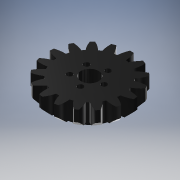
# Autodesk Inventor part: Spur Gear1
Saved by Autodesk Inventor 2017 (Build 210142000, 142)
## iProperties
Created: 2019-10-27
Part Number: Spur Gear1
Material: ABS Plastic
Document SubType Name: Modeling
Designer: Zach
Categories: <?xml version="1.0" encoding="UTF-16"?> <MemberInstance><Categories><FamilyTemplate><FamilyTemplateParameter ValueType="xs:double" Id="1" ObjectReferenceKey="da_z" ObjectType="kUserParameterObject"/><FamilyTemplateParameter ValueType="xs:double" Id="2" ObjectReferenceKey="da_b" ObjectType="kUserParameterObject"/><FamilyTemplateParameter ValueType="xs:double" Id="3" ObjectReferenceKey="da_beta" ObjectType="kUserParameterObject"/><FamilyTemplateParameter ValueType="xs:double" Id="4" ObjectReferenceKey="da_da" ObjectType="kUserParameterObject"/><FamilyTemplateParameter ValueType="xs:double" Id="5" ObjectReferenceKey="da_aw" ObjectType="kUserParameterObject"/><FamilyTemplateParameter ValueType="xs:string" Id="6" ObjectReferenceKey="EAIAABAAAACIAQAAAAAAAIAAAAAAAAAA" ObjectType="83910656" SubObjectId="SurfaceGeometry"/></FamilyTemplate><ParamToTemplateMap><ParamToTemplate CategoryParameter="//CategoryParameter[@InternalName='046C89C9-8512-4d59-83FE-43B91F4F132A']" TemplateParameter="1"/><ParamToTemplate CategoryParameter="//CategoryParameter[@InternalName='2552DF32-E462-4b46-AEBF-C6C7768E72AC']" TemplateParameter="2"/><ParamToTemplate CategoryParameter="//CategoryParameter[@InternalName='C9EE641D-15FC-4fae-A226-E94C4372FDD7']" TemplateParameter="3"/><ParamToTemplate><ParamToTemplate CategoryParameter="//CategoryParameter[@InternalName='00B6519A-459B-49c7-AD84-2E56D39A5744']" ConstantValue="0.000000"/></ParamToTemplate><ParamToTemplate><ParamToTemplate CategoryParameter="//CategoryParameter[@InternalName='04B31F0E-C7A6-4894-AA32-9629BEFACF47']" ConstantValue="1.000000"/></ParamToTemplate><ParamToTemplate><ParamToTemplate CategoryParameter="//CategoryParameter[@InternalName='43CBEC2E-7847-49e7-A936-2F7889FCB2D9']" ConstantValue="0.250000"/></ParamToTemplate><ParamToTemplate><ParamToTemplate CategoryParameter="//CategoryParameter[@InternalName='B1EFC894-105D-4ebd-86BF-FA20ED196853']" ConstantValue="0.350000"/></ParamToTemplate><ParamToTemplate><ParamToTemplate CategoryParameter="//CategoryParameter[@InternalName='51175063-3D10-4879-93E8-6246FE8B403D']" ConstantValue="2060000000.000000"/></ParamToTemplate><ParamToTemplate><ParamToTemplate CategoryParameter="//CategoryParameter[@InternalName='A3A52E27-4454-46a9-B0BD-C932399B70AF']" ConstantValue="0.300000"/></ParamToTemplate><ParamToTemplate><ParamToTemplate CategoryParameter="//CategoryParameter[@InternalName='91B76062-C214-41d9-B1B9-14D2AB99603D']" ConstantValue="0.200000"/></ParamToTemplate><ParamToTemplate><ParamToTemplate CategoryParameter="//CategoryParameter[@InternalName='374E806E-8B8A-4dda-A9AA-1039D6500AD2']" ConstantValue="5.000000"/></ParamToTemplate><ParamToTemplate><ParamToTemplate CategoryParameter="//CategoryParameter[@InternalName='2D373A89-B862-43d6-8D0B-0CBF12AB9F6C']" ConstantValue="0.392699"/></ParamToTemplate><ParamToTemplate CategoryParameter="//CategoryParameter[@InternalName='37777632-D6A2-4fac-9D53-DB8ACD95C989']" TemplateParameter="4"/><ParamToTemplate CategoryParameter="//CategoryParameter[@InternalName='FD1017F1-B727-4f7e-9707-0F86F1FF9423']" TemplateParameter="5"/><ParamToTemplate><ParamToTemplate CategoryParameter="//CategoryParameter[@InternalName='9E1B4470-B2D3-4ff1-B813-535BB4CDF51A']" ConstantValue="3520000.000000"/></ParamToTemplate><ParamToTemplate><ParamToTemplate CategoryParameter="//CategoryParameter[@InternalName='F8452263-BFF6-458c-9FB1-07C4B99E95CD']" ConstantValue="11400000.000000"/></ParamToTemplate><ParamToTemplate><ParamToTemplate CategoryParameter="//CategoryParameter[@InternalName='3E3BB259-FD49-497f-8171-6EBC954A3479']" ConstantValue="2.000000"/></ParamToTemplate><ParamToTemplate CategoryParameter="//CategoryParameter[@InternalName='27C3BAF2-7550-4e4b-AE2C-0DB134B7D9B7']" TemplateParameter="6"/></ParamToTemplateMap><Category DisplayName="Gear" InternalName="DC85795E-93AB-48d5-8EEE-5A27447B64BD" Mnemonic="Gear"><CategoryParameter DisplayName="z" InternalName="046C89C9-8512-4d59-83FE-43B91F4F132A" Mnemonic="z"/><CategoryParameter DisplayName="b" InternalName="2552DF32-E462-4b46-AEBF-C6C7768E72AC" Mnemonic="b"/><CategoryParameter DisplayName="||b|" InternalName="C9EE641D-15FC-4fae-A226-E94C4372FDD7" Mnemonic="beta"/><CategoryParameter DisplayName="x" InternalName="00B6519A-459B-49c7-AD84-2E56D39A5744" Mnemonic="x"/><CategoryParameter DisplayName="a*" InternalName="04B31F0E-C7A6-4894-AA32-9629BEFACF47" Mnemonic="a"/><CategoryParameter DisplayName="c*" InternalName="43CBEC2E-7847-49e7-A936-2F7889FCB2D9" Mnemonic="c"/><CategoryParameter DisplayName="r|.f|*" InternalName="B1EFC894-105D-4ebd-86BF-FA20ED196853" Mnemonic="rf"/><CategoryParameter DisplayName="E" InternalName="51175063-3D10-4879-93E8-6246FE8B403D" Mnemonic="E"/><CategoryParameter DisplayName="||m|" InternalName="A3A52E27-4454-46a9-B0BD-C932399B70AF" Mnemonic="mi"/><Category DisplayName="SpurGear" InternalName="26C5A22E-A91E-4dfd-A3B3-23CCAFAE1764" Mnemonic="SpurGear"><CategoryParameter DisplayName="m" InternalName="91B76062-C214-41d9-B1B9-14D2AB99603D" Mnemonic="m"/><CategoryParameter DisplayName="P" InternalName="374E806E-8B8A-4dda-A9AA-1039D6500AD2" Mnemonic="PP"/><CategoryParameter DisplayName="||a|" InternalName="2D373A89-B862-43d6-8D0B-0CBF12AB9F6C" Mnemonic="alpha"/><CategoryParameter DisplayName="d|.a|" InternalName="37777632-D6A2-4fac-9D53-DB8ACD95C989" Mnemonic="da"/><CategoryParameter DisplayName="a|.w|" InternalName="FD1017F1-B727-4f7e-9707-0F86F1FF9423" Mnemonic="aw"/><CategoryParameter DisplayName="||s||.Flim|" InternalName="9E1B4470-B2D3-4ff1-B813-535BB4CDF51A" Mnemonic="sFlim"/><CategoryParameter DisplayName="||s||.Hlim|" InternalName="F8452263-BFF6-458c-9FB1-07C4B99E95CD" Mnemonic="sHlim"/><CategoryParameter DisplayName="type" InternalName="3E3BB259-FD49-497f-8171-6EBC954A3479" Mnemonic="type"/><CategoryParameter DisplayName="PitchDiameter" InternalName="27C3BAF2-7550-4e4b-AE2C-0DB134B7D9B7" Mnemonic="IDS_PITCHDIAM"/></Category></Category></Categories></MemberInstance>
Density: 1.06 g/cm^3
Appearance: Smooth - Black
CustomPartVersion: 1
Author: Zach
Autodesk Inventor part; units mm, degrees
sketch "Sketch1" plane through (0, 0, 0) normal (0, 0, 1) x (1, 0, 0)
  circle A0 centre (0, 0) radius 19
  dimension "d0" = 38
  constraints: 1 centre point
  measures "d0" diameter of A0
extrude "Extrusion1" add sketch "Sketch1" along normal blind 8
ref_plane "Work Plane2" through (0, 0, 4) normal (0, 0, 1) x (1, 0, 0)
sketch "Sketch2" plane through (0, 0, 0) normal (0, 0, -1) x (-1, 0, 0)
  circle A0 centre (0, 0) radius 19 projected
  circle A1 centre (0, 0) radius 17
  dimension "d3" = 34
  constraints: 1 centre point, 1 coincident
  measures "d3" diameter of A1
surface extrude "Pitch Diameter" sketch "Sketch2" against normal through all shown no curves A1
ref_plane "Work Plane8" through (0, 0, 0) normal (0.9829731, 0.1837495, 0) x (0, 0, 1)
ref_plane "Work Plane9" through (0, 0, 0) normal (1, 0, 0) x (0, 1, 0)
spur gear teeth "Spur Gear" teeth 17 pitch diameter 34 tip diameter 38 root diameter 29 face width 8 start plane through (0, 0, 0) normal (0, 0, -1) x (-1, 0, 0)
sketch "Sketch3" plane through (0, 0, 8) normal (0, 0, 1) x (1, 0, 0)
  circle A0 centre (0, 0) radius 4
  circle A1 centre (6.5, 0) radius 1.25
  circle A2 centre (2.0086, 6.1819) radius 1.25
  circle A3 centre (-5.2586, 3.8206) radius 1.25
  circle A4 centre (-5.2586, -3.8206) radius 1.25
  circle A5 centre (2.0086, -6.1819) radius 1.25
  dimension "d49" = 8
  dimension "d50" = 2.5
  dimension "d51" = 6.5
  dimension "d54" = 360
  constraints: 6 centre point, 1 coincident, 1 horizontal alignment, 11 other
  measures "d49" diameter of A0
  measures "d50" diameter of A1
  measures "d51" distance of A1.centre point (0, 0)
extrude "Extrusion2" cut sketch "Sketch3" against normal through all
sketch "Sketch4" plane through (0, 0, 0) normal (0, 0, -1) x (-1, 0, 0)
  circle A0 centre (0, 0) radius 11.5
  circle A1 centre (-2.0086, -6.1819) radius 1.25 projected
  circle A2 centre (5.2586, 3.8206) radius 1.25 projected
  circle A3 centre (-6.5, 0) radius 1.25 projected
  circle A4 centre (-2.0086, 6.1819) radius 1.25 projected
  circle A5 centre (5.2586, -3.8206) radius 1.25 projected
  circle A6 centre (0, 0) radius 4 projected
  arc A7 (0.8775, 18.9797) -> (-0.8775, 18.9797) centre (0, 0) ccw projected
  arc A8 (6.038, 18.0151) -> (3.3198, 14.1149) centre (16.9951, 7.4811) ccw projected
  arc A9 (3.3198, 14.1149) -> (2.0033, 14.361) centre (0, 0) ccw projected
  arc A10 (2.0033, 14.361) -> (0.8775, 18.9797) centre (-13.145, 13.1153) ccw projected
  arc A11 (-0.8775, 18.9797) -> (-2.0033, 14.361) centre (13.145, 13.1153) ccw projected
  arc A12 (-2.0033, 14.361) -> (-3.3198, 14.1149) centre (0, 0) ccw projected
  arc A13 (-3.3198, 14.1149) -> (-6.038, 18.0151) centre (-16.9951, 7.4811) ccw projected
  arc A14 (-6.038, 18.0151) -> (-7.6745, 17.3811) centre (0, 0) ccw projected
  arc A15 (-7.6745, 17.3811) -> (-7.0558, 12.6675) centre (7.5195, 16.9782) ccw projected
  arc A16 (-7.0558, 12.6675) -> (-8.1945, 11.9625) centre (0, 0) ccw projected
  arc A17 (-8.1945, 11.9625) -> (-12.1381, 14.6173) centre (-18.55, 0.8366) ccw projected
  arc A18 (-12.1381, 14.6173) -> (-13.435, 13.435) centre (0, 0) ccw projected
  arc A19 (-13.435, 13.435) -> (-11.1553, 9.2633) centre (0.8785, 18.548) ccw projected
  arc A20 (-11.1553, 9.2633) -> (-11.9625, 8.1945) centre (0, 0) ccw projected
  arc A21 (-11.9625, 8.1945) -> (-16.5988, 9.2455) centre (-17.5996, -5.9209) ccw projected
  arc A22 (-16.5988, 9.2455) -> (-17.3811, 7.6745) centre (0, 0) ccw projected
  arc A23 (-17.3811, 7.6745) -> (-13.7483, 4.608) centre (-5.8811, 17.6129) ccw projected
  arc A24 (-13.7483, 4.608) -> (-14.1149, 3.3198) centre (0, 0) ccw projected
  arc A25 (-14.1149, 3.3198) -> (-18.8178, 2.625) centre (-14.2722, -11.8788) ccw projected
  arc A26 (-18.8178, 2.625) -> (-18.9797, 0.8775) centre (0, 0) ccw projected
  arc A27 (-18.9797, 0.8775) -> (-14.4845, -0.6697) centre (-11.8465, 14.299) ccw projected
  arc A28 (-14.4845, -0.6697) -> (-14.361, -2.0033) centre (0, 0) ccw projected
  arc A29 (-14.361, -2.0033) -> (-18.4953, -4.3501) centre (-9.0173, -16.2323) ccw projected
  arc A30 (-18.4953, -4.3501) -> (-18.0151, -6.038) centre (0, 0) ccw projected
  arc A31 (-18.0151, -6.038) -> (-13.2645, -5.8569) centre (-16.2119, 9.054) ccw projected
  arc A32 (-13.2645, -5.8569) -> (-12.6675, -7.0558) centre (0, 0) ccw projected
  arc A33 (-12.6675, -7.0558) -> (-15.675, -10.7376) centre (-2.5446, -18.3936) ccw projected
  arc A34 (-15.675, -10.7376) -> (-14.6173, -12.1381) centre (0, 0) ccw projected
  arc A35 (-14.6173, -12.1381) -> (-10.253, -10.253) centre (-18.3879, 2.5862) ccw projected
  arc A36 (-10.253, -10.253) -> (-9.2633, -11.1553) centre (0, 0) ccw projected
  arc A37 (-9.2633, -11.1553) -> (-10.7376, -15.675) centre (4.2718, -18.0708) ccw projected
  arc A38 (-10.7376, -15.675) -> (-9.2455, -16.5988) centre (0, 0) ccw projected
  arc A39 (-9.2455, -16.5988) -> (-5.8569, -13.2645) centre (-18.0804, -4.2309) ccw projected
  arc A40 (-5.8569, -13.2645) -> (-4.608, -13.7483) centre (0, 0) ccw projected
  arc A41 (-4.608, -13.7483) -> (-4.3501, -18.4953) centre (10.5112, -15.3074) ccw projected
  arc A42 (-4.3501, -18.4953) -> (-2.625, -18.8178) centre (0, 0) ccw projected
  arc A43 (-2.625, -18.8178) -> (-0.6697, -14.4845) centre (-15.3311, -10.4766) ccw projected
  arc A44 (-0.6697, -14.4845) -> (0.6697, -14.4845) centre (0, 0) ccw projected
  arc A45 (0.6697, -14.4845) -> (2.625, -18.8178) centre (15.3311, -10.4766) ccw projected
  arc A46 (2.625, -18.8178) -> (4.3501, -18.4953) centre (0, 0) ccw projected
  arc A47 (4.3501, -18.4953) -> (4.608, -13.7483) centre (-10.5112, -15.3074) ccw projected
  arc A48 (4.608, -13.7483) -> (5.8569, -13.2645) centre (0, 0) ccw projected
  arc A49 (5.8569, -13.2645) -> (9.2455, -16.5988) centre (18.0804, -4.2309) ccw projected
  arc A50 (9.2455, -16.5988) -> (10.7376, -15.675) centre (0, 0) ccw projected
  arc A51 (10.7376, -15.675) -> (9.2633, -11.1553) centre (-4.2718, -18.0708) ccw projected
  arc A52 (9.2633, -11.1553) -> (10.253, -10.253) centre (0, 0) ccw projected
  arc A53 (10.253, -10.253) -> (14.6173, -12.1381) centre (18.3879, 2.5862) ccw projected
  arc A54 (14.6173, -12.1381) -> (15.675, -10.7376) centre (0, 0) ccw projected
  arc A55 (15.675, -10.7376) -> (12.6675, -7.0558) centre (2.5446, -18.3936) ccw projected
  arc A56 (12.6675, -7.0558) -> (13.2645, -5.8569) centre (0, 0) ccw projected
  arc A57 (13.2645, -5.8569) -> (18.0151, -6.038) centre (16.2119, 9.054) ccw projected
  arc A58 (18.0151, -6.038) -> (18.4953, -4.3501) centre (0, 0) ccw projected
  arc A59 (18.4953, -4.3501) -> (14.361, -2.0033) centre (9.0173, -16.2323) ccw projected
  arc A60 (14.361, -2.0033) -> (14.4845, -0.6697) centre (0, 0) ccw projected
  arc A61 (14.4845, -0.6697) -> (18.9797, 0.8775) centre (11.8465, 14.299) ccw projected
  arc A62 (18.9797, 0.8775) -> (18.8178, 2.625) centre (0, 0) ccw projected
  arc A63 (18.8178, 2.625) -> (14.1149, 3.3198) centre (14.2722, -11.8788) ccw projected
  arc A64 (14.1149, 3.3198) -> (13.7483, 4.608) centre (0, 0) ccw projected
  arc A65 (13.7483, 4.608) -> (17.3811, 7.6745) centre (5.8811, 17.6129) ccw projected
  arc A66 (17.3811, 7.6745) -> (16.5988, 9.2455) centre (0, 0) ccw projected
  arc A67 (16.5988, 9.2455) -> (11.9625, 8.1945) centre (17.5996, -5.9209) ccw projected
  arc A68 (11.9625, 8.1945) -> (11.1553, 9.2633) centre (0, 0) ccw projected
  arc A69 (11.1553, 9.2633) -> (13.435, 13.435) centre (-0.8785, 18.548) ccw projected
  arc A70 (13.435, 13.435) -> (12.1381, 14.6173) centre (0, 0) ccw projected
  arc A71 (12.1381, 14.6173) -> (8.1945, 11.9625) centre (18.55, 0.8366) ccw projected
  arc A72 (8.1945, 11.9625) -> (7.0558, 12.6675) centre (0, 0) ccw projected
  arc A73 (7.0558, 12.6675) -> (7.6745, 17.3811) centre (-7.5195, 16.9782) ccw projected
  arc A74 (7.6745, 17.3811) -> (6.038, 18.0151) centre (0, 0) ccw projected
  dimension "d58" = 23
  constraints: 1 centre point, 1 coincident
  measures "d58" diameter of A0
extrude "Extrusion3" add sketch "Sketch4" along normal blind 3 contours A0
chamfer "Chamfer1" distance 3 angle 45 17 edges at (15.1623, -11.4501, 0) (18.2747, -5.1996, 0) (18.9189, 1.7531, 0) (17.0081, 8.469, 0) (12.8002, 14.0412, 0) (6.8636, 17.717, 0) (0, 19, 0) (-6.8636, 17.717, 0) (-12.8002, 14.0412, 0) (-17.0081, 8.469, 0) (-18.9189, 1.7531, 0) (-18.2747, -5.1996, 0) (-15.1623, -11.4501, 0) (-10.0022, -16.1541, 0) (-3.4912, -18.6765, 0) (3.4912, -18.6765, 0) (10.0022, -16.1541, 0)
equation "\"d0\" = da_da"
equation "\"d1\" = da_b"
equation "\"d3\" = da_dw"
equation "\"d16\" = da_aw"
equation "\"d43\" = da_aw"
equation "\"d46\" = da_aw"
equation "\"da_da\" = 38"
equation "\"da_b\" = 8"
equation "\"da_dw\" = 34"
equation "\"da_aw\" = 35"
body "Solid1"
body "Srf1"
